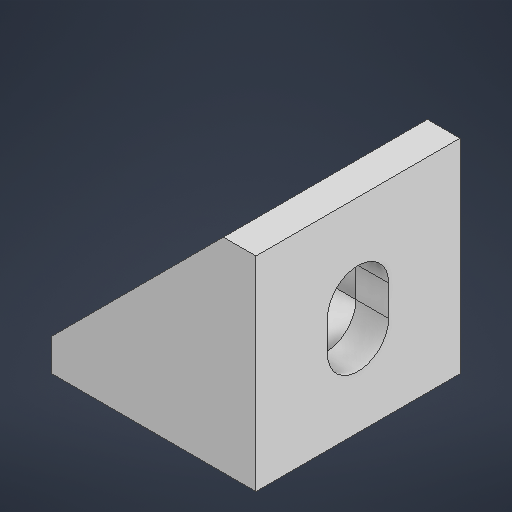
# Autodesk Inventor part: Al_Bracket
Saved by Autodesk Inventor 2026.2 (Build 302298010, 298A)
## iProperties
Created: 2026-08-19
Part Number: Al_Bracket
Material: Generic
Document SubType Name: Modeling
Designer: aiden
Density: 1 g/cm^3
Appearance: Default
Author: aiden
Autodesk Inventor part; units mm, degrees
ref_plane "YZ Plane" through (0, 0, 0) normal (1, 0, 0) x (0, 1, 0)
ref_plane "XZ Plane" through (0, 0, 0) normal (0, 1, 0) x (-1, 0, 0)
ref_plane "XY Plane" through (0, 0, 0) normal (0, 0, 1) x (1, 0, 0)
sketch "Sketch1" plane through (0, 0, 0) normal (0, 1, 0) x (-1, 0, 0)
  line L0 (0, 0) -> (20, 0)
  line L1 (20, 0) -> (20, -20)
  line L2 (20, -20) -> (0, -20)
  line L3 (0, -20) -> (0, 0)
  dimension "d0" = 20
  dimension "d1" = 20
  constraints: 8 end point, 2 parallel, 1 horizontal, 1 perpendicular
  measures "d0" distance of L1.end L2.end
  measures "d1" distance of L0.end L1.end
extrude "Extrusion1" add sketch "Sketch1" along normal blind 20
sketch "Sketch2" plane through (-20, 0, 0) normal (0, 0, 1) x (1, 0, 0)
  line L0 (20, 0) -> (0, 0) projected
  line L1 (20, 0) -> (20, 20) projected
  line L2 (20, 20) -> (0, 20) projected
  line L3 (0, 20) -> (16.8, 20)
  line L4 (0, 0) -> (0, 20) projected
  line L5 (1.6773, 3.2839) -> (0, 3.1156)
  line L6 (0, 20) -> (0, 3.2)
  line L7 (16.8, 20) -> (0, 3.2)
  dimension "d6" = 16.8
  dimension "d9" = 16.8
  constraints: 8 end point, 3 point on line
  measures "d6" distance of L2.end L3.end
  measures "d9" distance of L2.end L6.end
extrude "Extrusion3" cut sketch "Sketch2" against normal blind 20 contours L7 L4 L2
sketch "Sketch3" plane through (0, 20, 0) normal (0, 1, 0) x (1, 0, 0)
  line L0 (0, 18) -> (-20, 18)
  line L1 (-20, 18) -> (-20, 2)
  line L2 (-20, 2) -> (0, 2)
  line L3 (0, 2) -> (0, 18)
  line L4 (-20, 20) -> (-3.2, 20) projected
  line L5 (-4, 18) -> (12, 18) construction
  line L6 (0, 18) -> (0, 2)
  line L7 (-3.2, 18) -> (-3.2, 2)
  point P0 (-20, 10)
  dimension "d12" = 16
  dimension "d13" = 2
  constraints: 14 end point, 3 perpendicular, 3 point on line, 2 horizontal, 2 parallel, 1 midpoint
  measures "d12" distance of L1.end L0.end
  measures "d13" distance between parallel lines of L4 L0
extrude "Extrusion4" cut sketch "Sketch3" against normal blind 16.8 contours L7 L2 L1 L0
sketch "Sketch4" plane through (0, 3.2, 0) normal (0, 1, 0) x (1, 0, 0)
  line L0 (-14.2, 13) -> (-5.2, 13)
  line L1 (-5.2, 13) -> (-5.2, 7)
  line L2 (-5.2, 7) -> (-14.2, 7)
  line L3 (-14.2, 7) -> (-14.2, 13)
  line L4 (-3.2, 18) -> (-3.2, 2) projected
  arc A0 (-8.2, 7) -> (-8.2, 13) centre (-8.2, 10) ccw
  line L5 (-18, 13.026) -> (-18, 7.026)
  line L6 (-20, 2) -> (-20, 18) projected
  ellipse E0 centre (-14.2, 10) end of major axis (-18, 10) minor radius 3 (-14.2, 13) -> (-14.2, 7) ccw
  arc A1 (-11.2, 13) -> (-11.2, 7) centre (-11.2, 10) ccw
  line L7 (-5.2, 10) -> (-18, 10)
  line L8 (-20, 18) -> (-3.2, 18) projected
  point P0 (0, 0)
  dimension "d18" = 6
  dimension "d19" = 9
  dimension "d20" = 2
  dimension "d21" = 6
  dimension "d22" = 2
  dimension "d40" = 8
  constraints: 12 end point, 6 tangent, 5 point on circle, 5 point on line, 2 centre point, 2 parallel, 1 horizontal, 1 midpoint, 1 perpendicular, 1 vertical, 5 other
  measures "d18" distance of L0.end L1.end
  measures "d19" distance of L1.end L2.end
  measures "d20" distance between parallel lines of L4 L1
  measures "d21" distance of L5.start L5.end
  measures "d22" distance between parallel lines of L5 L6
  measures "d40" distance between parallel lines of L8 L7
extrude "Extrusion5" cut sketch "Sketch4" against normal blind 16.8 contours L0 A0 L7 A1 | L7 A0 L2 A1
sketch "Sketch8" plane through (-3.2, 0.3648, -21.4635) normal (-1, 0, 0) x (0, -1, 0)
  line L0 (-13.8352, 14.4635) -> (-4.8352, 14.4635)
  line L1 (-4.8352, 14.4635) -> (-4.8352, 8.4635)
  line L2 (-4.8352, 8.4635) -> (-13.8352, 8.4635)
  line L3 (-13.8352, 8.4635) -> (-13.8352, 14.4635)
  line L4 (-2.8352, 18) -> (-2.8352, 2)
  arc A0 (-7.8352, 8.4635) -> (-7.8352, 14.4635) centre (-7.8352, 11.4635) ccw
  line L5 (-18, 13.026) -> (-18, 7.026)
  line L6 (-20, 2) -> (-20, 18)
  ellipse E0 centre (-13.8352, 11.4635) end of major axis (-18, 11.4635) minor radius 3 (-13.8352, 14.4635) -> (-13.8352, 8.4635) ccw
  arc A1 (-10.8352, 14.4635) -> (-10.8352, 8.4635) centre (-10.8352, 11.4635) ccw
  line L7 (-4.8352, 11.4635) -> (-18, 11.4635)
  line L8 (-2.8352, 19.4635) -> (-2.8352, 3.4635) projected
  line L9 (-19.6352, 19.4635) -> (-2.8352, 19.4635) projected
  point P0 (0, 0)
  dimension "d34" = 6
  dimension "d33" = 9
  dimension "d32" = 2
  dimension "d31" = 6
  dimension "d30" = 2
  dimension "d38" = 0
  dimension "d39" = 5
  constraints: 16 end point, 6 tangent, 5 point on circle, 5 point on line, 2 centre point, 2 parallel, 1 horizontal, 1 midpoint, 1 perpendicular, 1 vertical, 5 other
  measures "d34" distance of L0.end L1.end
  measures "d33" distance of L1.end L2.end
  measures "d32" distance between parallel lines of L4 L1
  measures "d31" distance of L5.start L5.end
  measures "d30" distance between parallel lines of L5 L6
  measures "d38" distance between parallel lines of L4 L8
  measures "d39" distance between parallel lines of L9 L0
extrude "Extrusion7" cut sketch "Sketch8" against normal blind 16.8 contours L0 A0 L7 A1 | L7 A0 L2 A1
body "Solid1"
